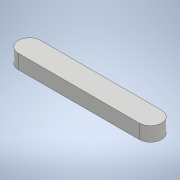
# Autodesk Inventor part: 零件2
Saved by Autodesk Inventor 2020 (Build 240168000, 168)
## iProperties
Created: 2021-06-22
Part Number: 零件2
Material: 常规
Document SubType Name: Modeling
Designer: dell
Density: 1 g/cm^3
Appearance: 默认
Author: dell
Autodesk Inventor part; units mm, degrees
ref_plane "YZ Plane" through (0, 0, 0) normal (1, 0, 0) x (0, 1, 0)
ref_plane "XZ Plane" through (0, 0, 0) normal (0, 1, 0) x (-1, 0, 0)
ref_plane "XY Plane" through (0, 0, 0) normal (0, 0, 1) x (1, 0, 0)
sketch "草图1" plane through (0, 0, 0) normal (0, 0, 1) x (1, 0, 0)
  line L0 (-45, 7) -> (45, 7) projected
  arc A0 (-45, 7) -> (-45, -7) centre (-45, 0) ccw projected
  line L1 (45, -7) -> (-45, -7) projected
  arc A1 (45, -7) -> (45, 7) centre (45, 0) ccw projected
  line L2 (-38, 0) -> (38, 0) construction
  line L3 (-38, -7) -> (38, -7)
  line L4 (38, 7) -> (-38, 7)
  arc A2 (-38, 7) -> (-38, -7) centre (-38, 0) ccw
  arc A3 (38, -7) -> (38, 7) centre (38, 0) ccw
  line L5 (0, 9.8) -> (0, -9.8) projected
  point P0 (0, 0)
  dimension "d2" = 90
  dimension "d3" = 7
  constraints: 8 end point, 4 point on circle, 4 tangent, 2 centre point, 1 horizontal, 1 horizontal alignment, 1 midpoint, 1 parallel, 1 symmetric about line
  measures "d3" radius of A2
extrude "拉伸2" add sketch "草图1" along normal blind 9 contours L0 L5 L1 A2 | L0 A3 L1 L5
